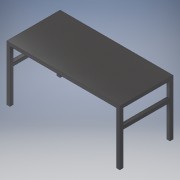
# Autodesk Inventor part: bottomtable
Saved by Autodesk Inventor 2017 (Build 210142000, 142)
## iProperties
Created: 2018-08-24
Part Number: bottomtable
Material: Generic
Document SubType Name: Modeling
Designer: emmacarlisle
Density: 1 g/cm^3
Appearance: Machined 02
Author: emmacarlisle
Autodesk Inventor part; units mm, degrees
ref_plane "YZ Plane" through (0, 0, 0) normal (1, 0, 0) x (0, 1, 0)
ref_plane "XZ Plane" through (0, 0, 0) normal (0, 1, 0) x (-1, 0, 0)
ref_plane "XY Plane" through (0, 0, 0) normal (0, 0, 1) x (1, 0, 0)
sketch "Sketch1" plane through (0, 0, 0) normal (0, 0, 1) x (1, 0, 0)
  line L0 (0, 0) -> (1420, 0)
  line L1 (1420, 0) -> (1420, 695)
  line L2 (1420, 695) -> (0, 695)
  line L3 (0, 695) -> (0, 0)
  dimension "d0" = 695
  dimension "d1" = 1420
  constraints: 8 end point, 2 parallel, 1 horizontal, 1 perpendicular
  measures "d0" distance of L0.end L1.end
  measures "d1" distance of L1.end L2.end
extrude "Extrusion1" add sketch "Sketch1" along normal blind 670
sketch "Sketch2" plane through (1420, 0, 0) normal (1, 0, 0) x (0, 0, -1)
  line L0 (-630, 0) -> (-40, 0)
  line L1 (-40, 0) -> (-40, 420)
  line L2 (-40, 420) -> (-630, 420)
  line L3 (-630, 420) -> (-630, 0)
  line L4 (-670, 695) -> (-670, 0) projected
  line L5 (0, 0) -> (0, 695) projected
  line L6 (0, 0) -> (-670, 0) projected
  dimension "d4" = 420
  dimension "d5" = 40
  dimension "d6" = 40
  constraints: 8 end point, 2 parallel, 1 horizontal, 1 perpendicular, 1 point on line
  measures "d4" distance of L2.end L0.start
  measures "d5" distance between parallel lines of L4 L3
  measures "d6" distance between parallel lines of L5 L1
extrude "Extrusion2" cut sketch "Sketch2" against normal blind 2000
sketch "Sketch3" plane through (1420, 0, 0) normal (1, 0, 0) x (0, 0, -1)
  line L0 (-630, 460) -> (-40, 460)
  line L1 (-40, 460) -> (-40, 655)
  line L2 (-40, 655) -> (-630, 655)
  line L3 (-630, 655) -> (-630, 460)
  line L4 (0, 695) -> (-670, 695) projected
  line L5 (-670, 695) -> (-670, 0) projected
  line L6 (-630, 420) -> (-40, 420) projected
  line L7 (0, 0) -> (0, 695) projected
  dimension "d9" = 40
  dimension "d10" = 40
  dimension "d11" = 40
  dimension "d12" = 40
  constraints: 8 end point, 2 parallel, 1 horizontal, 1 perpendicular
  measures "d9" distance between parallel lines of L4 L2
  measures "d10" distance between parallel lines of L5 L3
  measures "d11" distance between parallel lines of L0 L6
  measures "d12" distance between parallel lines of L7 L1
extrude "Extrusion3" cut sketch "Sketch3" against normal blind 2000
sketch "Sketch4" plane through (0, 0, 670) normal (0, 0, 1) x (1, 0, 0)
  line L0 (40, 0) -> (1380, 0)
  line L1 (1380, 0) -> (1380, 655)
  line L2 (1380, 655) -> (40, 655)
  line L3 (40, 655) -> (40, 0)
  line L4 (0, 0) -> (1420, 0) projected
  line L5 (0, 420) -> (0, 0) projected
  line L6 (1420, 0) -> (1420, 695) projected
  line L7 (1420, 695) -> (0, 695) projected
  dimension "d15" = 40
  dimension "d16" = 40
  dimension "d17" = 40
  constraints: 8 end point, 2 parallel, 1 horizontal, 1 perpendicular, 1 point on line
  measures "d15" distance between parallel lines of L5 L3
  measures "d16" distance between parallel lines of L6 L1
  measures "d17" distance between parallel lines of L7 L2
extrude "Extrusion4" cut sketch "Sketch4" against normal blind 1000
body "Solid1"
